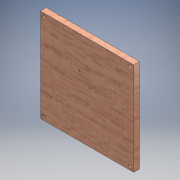
# Autodesk Inventor part: support_balise
Saved by Autodesk Inventor 2017 (Build 210142000, 142)
## iProperties
Created: 2017-04-21
Part Number: support_balise
Material: Generic
Document SubType Name: Modeling
Designer: franc
Density: 1 g/cm^3
Appearance: Default
Author: franc
Autodesk Inventor part; units mm, degrees
ref_plane "YZ Plane" through (0, 0, 0) normal (1, 0, 0) x (0, 1, 0)
ref_plane "XZ Plane" through (0, 0, 0) normal (0, 1, 0) x (-1, 0, 0)
ref_plane "XY Plane" through (0, 0, 0) normal (0, 0, 1) x (1, 0, 0)
sketch "Sketch1" plane through (0, 0, 0) normal (0, 1, 0) x (-1, 0, 0)
  line L0 (2.5145, 3.569) -> (-77.4855, 3.569)
  line L1 (-77.4855, 3.569) -> (-77.4855, -76.431)
  line L2 (-77.4855, -76.431) -> (2.5145, -76.431)
  line L3 (2.5145, -76.431) -> (2.5145, 3.569)
  circle A0 centre (-0.4855, 0.569) radius 1.5
  circle A1 centre (-0.4855, -73.431) radius 1.5
  circle A2 centre (-74.4855, 0.569) radius 1.5
  circle A3 centre (-74.4855, -73.431) radius 1.5
  point P0 (0, 0)
  dimension "d0" = 80
  dimension "d1" = 80
  dimension "d4" = 3
  dimension "d5" = 3
  dimension "d6" = 3
  dimension "d7" = 3
  dimension "d8" = 3
  dimension "d9" = 3
  dimension "d10" = 3
  dimension "d11" = 3
  dimension "d12" = 3
  dimension "d13" = 3
  dimension "d14" = 3
  dimension "d15" = 3
  constraints: 8 end point, 4 centre point, 2 parallel, 1 horizontal, 1 perpendicular
  measures "d0" distance of L2.end L0.start
  measures "d1" distance of L0.start L0.end
  measures "d4" diameter of A0
  measures "d5" distance from line of L3 A0.centre
  measures "d6" distance from line of L0 A0.centre
  measures "d7" distance from line of A2.centre L0
  measures "d8" distance from line of L1 A2.centre
  measures "d9" diameter of A2
  measures "d10" distance from line of L1 A3.centre
  measures "d11" distance from line of L2 A3.centre
  measures "d12" diameter of A3
  measures "d13" distance from line of L3 A1.centre
  measures "d14" distance from line of L2 A1.centre
  measures "d15" diameter of A1
extrude "Extrusion1" add sketch "Sketch1" along normal blind 5
body "Solid1"
